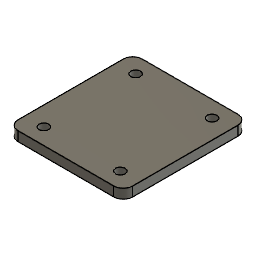
karetka_vertical (Autodesk Fusion 360 design; units mm, degrees)
Autodesk Fusion 360 part; units mm, degrees
sketch "Sketch1" plane through (0, 0, 0) normal (0, 1, 0) x (1, 0, 0)
  line L0 (30, -32.5) -> (-30, -32.5)
  line L1 (-30, -32.5) -> (-30, 32.5)
  line L2 (-30, 32.5) -> (30, 32.5)
  line L3 (30, 32.5) -> (30, -32.5)
  circle A0 centre (-20, 24) radius 2.5
  circle A1 centre (20, 24) radius 2.5
  line L4 (0, 0) -> (0, 5)
  line L5 (0, 0) -> (5, 0)
  circle A2 centre (-20, -24) radius 2.5
  circle A3 centre (20, -24) radius 2.5
  dimension "d1" = 60
  dimension "d2" = 65
  dimension "d5" = 5
  dimension "d6" = 5
  dimension "d13" = 24
  dimension "d14" = 24
  constraint horizontal L0
  constraint perpendicular L0 L1
  constraint parallel L0 L2
  constraint parallel L1 L3
  constraint coincident L4.start L5.start
  constraint vertical L4
  constraint perpendicular L4 L5
  constraint symmetric A0 L5 A2
  constraint symmetric A1 L5 A3
  measures "d1" distance of L1.end L2.end
  measures "d2" distance of L0.end L1.end
  measures "d5" diameter of A0
  measures "d6" diameter of A1
  measures "d13" vertical distance of L4.start A0.centre
  measures "d14" distance of A1.centre L5
extrude "Extrude1" add sketch "Sketch1" along normal blind 5
fillet "Fillet1" radius 5 4 edges at (-30, 2.5, -32.5) (30, 2.5, -32.5) (-30, 2.5, 32.5) (30, 2.5, 32.5)
